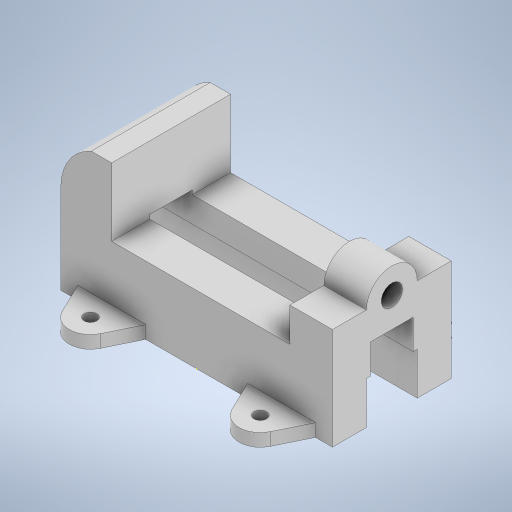
# Autodesk Inventor part: Pieza5-Tarea1
Saved by Autodesk Inventor 2024 (Build 280153000, 153)
## iProperties
Created: 2024-02-16
Part Number: Pieza5-Tarea1
Material: Genérico
Document SubType Name: Modeling
Designer: Diegolap
Density: 1 g/cm^3
Appearance: Valor por defecto
Mass: 816.406 g
Surface Area: 1054.14 cm^2
Volume: 816.406 cm^3
Author: Diegolap
Autodesk Inventor part; units mm, degrees
ref_plane "YZ Plane" through (0, 0, 0) normal (1, 0, 0) x (0, 1, 0)
ref_plane "XZ Plane" through (0, 0, 0) normal (0, 1, 0) x (-1, 0, 0)
ref_plane "XY Plane" through (0, 0, 0) normal (0, 0, 1) x (1, 0, 0)
sketch "Boceto1" plane through (0, 0, 0) normal (0, 1, 0) x (-1, 0, 0)
  line L0 (-101.6, 44.45) -> (101.6, 44.45)
  line L1 (101.6, 44.45) -> (101.6, -44.45)
  line L2 (101.6, -44.45) -> (-101.6, -44.45)
  line L3 (-101.6, -44.45) -> (-101.6, 44.45)
  line L4 (-101.6, 44.45) -> (101.6, -44.45) construction
  line L5 (101.6, 44.45) -> (-101.6, -44.45) construction
  point P0 (0, 0)
  dimension "d0" = 88.9
  dimension "d1" = 203.2
  constraints: 12 end point, 2 midpoint, 2 parallel, 1 horizontal, 1 perpendicular
  measures "d0" distance of L0.end L1.end
  measures "d1" distance of L0.start L0.end
extrude "Extrusión1" add sketch "Boceto1" along normal blind 50.8
sketch "Boceto2" plane through (0, 50.8, 0) normal (0, 1, 0) x (1, 0, 0)
  line L0 (101.6, 44.45) -> (-101.6, 44.45) projected
  line L1 (101.6, 44.45) -> (69.85, 44.45)
  line L2 (69.85, 44.45) -> (69.85, -44.45)
  line L3 (69.85, -44.45) -> (101.6, -44.45)
  line L4 (101.6, -44.45) -> (101.6, 44.45)
  point P0 (0, 0)
  dimension "d4" = 88.9
  dimension "d5" = 31.75
  constraints: 8 end point, 2 parallel, 1 horizontal, 1 perpendicular
  measures "d4" distance of L1.end L2.end
  measures "d5" distance of L2.end L3.end
extrude "Extrusión2" add sketch "Boceto2" along normal blind 25.4
sketch "Boceto3" plane through (101.6, 0, 44.45) normal (1, 0, 0) x (0, 0, -1)
  line L0 (0, 0) -> (0, 76.2) projected
  line L1 (0, 76.2) -> (88.9, 76.2) projected
  line L2 (0, 76.2) -> (88.9, 76.2)
  circle A0 centre (44.45, 76.2) radius 19.05
  circle A1 centre (44.45, 76.2) radius 7.9375
  point P0 (44.45, 0)
  dimension "d8" = 38.1
  dimension "d9" = 15.875
  constraints: 2 centre point, 2 end point, 1 coincident, 1 collinear, 1 midpoint
  measures "d8" diameter of A0
  measures "d9" diameter of A1
extrude "Extrusión3" add sketch "Boceto3" against normal blind 31.75 contours A1 L1 A0 | L1 A0 A1
sketch "Boceto4" plane through (101.6, 0, 44.45) normal (1, 0, 0) x (0, 0, -1)
  line L0 (52.3875, 76.2) -> (36.5125, 76.2) projected
  circle A0 centre (44.45, 76.2) radius 7.9375
  point P0 (44.45, 0)
  dimension "d12" = 15.875
  constraints: 1 centre point, 1 midpoint
  measures "d12" diameter of A0
extrude "Extrusión4" cut sketch "Boceto4" against normal blind 31.75
sketch "Boceto5" plane through (0, 50.8, 0) normal (0, 1, 0) x (1, 0, 0)
  line L0 (-101.6, -44.45) -> (101.6, -44.45) projected
  line L1 (-101.6, -44.45) -> (-63.5, -44.45)
  line L2 (-63.5, -44.45) -> (-63.5, 44.45)
  line L3 (-63.5, 44.45) -> (-101.6, 44.45)
  line L4 (-101.6, 44.45) -> (-101.6, -44.45)
  point P0 (0, 0)
  dimension "d15" = 38.1
  dimension "d16" = 88.9
  constraints: 8 end point, 2 parallel, 1 horizontal, 1 perpendicular
  measures "d15" distance of L2.end L3.end
  measures "d16" distance of L1.end L2.end
extrude "Extrusión5" add sketch "Boceto5" along normal blind 50.8
sketch "Boceto6" plane through (-101.6, 0, 44.45) normal (0, 0, 1) x (1, 0, 0)
  line L0 (0, 0) -> (0, 66.675)
  line L1 (0, 0) -> (0, 101.6) projected
  line L2 (38.1, 50.8) -> (38.1, 101.6) projected
  circle A0 centre (38.1, 66.675) radius 38.1
  line L3 (0, 66.675) -> (0, 101.6)
  line L4 (0, 101.6) -> (22.8732, 101.6)
  line L5 (0, 101.6) -> (38.1, 101.6) projected
  point P0 (101.6, 0)
  dimension "d20" = 76.2
  dimension "d19" = 66.675
  constraints: 6 end point, 3 point on line, 1 collinear, 3 other
  measures "d19" distance of L0.end L0.start
extrude "Extrusión6" cut sketch "Boceto6" against normal blind 101.6 contours L1 L4 A0
sketch "Boceto7" plane through (101.6, 0, 44.45) normal (1, 0, 0) x (0, 0, -1)
  line L0 (25.4, -31.75) -> (63.5, -31.75)
  line L1 (63.5, -31.75) -> (63.5, 31.75)
  line L2 (63.5, 31.75) -> (25.4, 31.75)
  line L3 (25.4, 31.75) -> (25.4, -31.75)
  line L4 (25.4, -31.75) -> (63.5, 31.75) construction
  line L5 (63.5, -31.75) -> (25.4, 31.75) construction
  line L6 (60.325, 53.975) -> (28.575, 53.975)
  line L7 (28.575, 53.975) -> (28.575, 31.75)
  line L8 (60.325, 31.75) -> (60.325, 53.975)
  line L9 (44.45, 31.75) -> (60.325, 53.975) construction
  line L10 (44.45, 31.75) -> (28.575, 53.975) construction
  point P0 (44.45, 0)
  dimension "d23" = 63.5
  dimension "d24" = 38.1
  dimension "d25" = 31.75
  dimension "d26" = 22.225
  dimension "d27" = 22.225
  dimension "d28" = 90
  dimension "d29" = 90
  constraints: 22 end point, 4 midpoint, 3 parallel, 2 point on line, 1 horizontal, 1 perpendicular
  measures "d23" distance of L0.end L1.end
  measures "d24" distance of L1.end L2.end
  measures "d25" distance of L6.start L6.end
  measures "d26" distance of L8.start L6.start
  measures "d27" distance of L6.end L7.end
  measures "d28" angle of L7 L6
  measures "d29" angle of L8 L6
extrude "Extrusión7" cut sketch "Boceto7" against normal blind 254
sketch "Boceto8" plane through (-101.6, 0, 44.45) normal (0, 0, 1) x (1, 0, 0)
  point P0 (101.6, 0)
sketch "Boceto9" plane through (0, 0, 0) normal (0, -1, 0) x (1, 0, 0)
  line L0 (-101.6, 44.45) -> (101.6, 44.45) projected
  line L1 (101.6, 44.45) -> (88.9, 44.45)
  line L2 (88.9, 44.45) -> (38.1, 44.45)
  line L3 (63.5, 44.45) -> (63.5, 60.325)
  circle A0 centre (63.5, 60.325) radius 4.7625
  circle A1 centre (63.5, 60.325) radius 15.875
  line L4 (38.1, 44.45) -> (49.2303, 67.2815)
  line L5 (88.9, 44.45) -> (77.7697, 67.2815)
  point P0 (0, 0)
  dimension "d32" = 12.7
  dimension "d33" = 50.8
  dimension "d34" = 15.875
  dimension "d35" = 9.525
  dimension "d36" = 31.75
  constraints: 10 end point, 2 centre point, 2 coincident, 2 point on circle, 2 point on line, 2 tangent, 1 midpoint, 1 vertical
  measures "d32" distance of L1.end L0.end
  measures "d33" distance of L2.end L1.end
  measures "d34" distance of L3.start L3.end
  measures "d35" diameter of A0
  measures "d36" diameter of A1
extrude "Extrusión8" add sketch "Boceto9" against normal blind 9.525
mirror "Simetría1" about plane through (0, 0, 0) normal (1, 0, 0) of "Extrusión8"
mirror "Simetría2" about plane through (0, 0, 0) normal (0, 0, 1) of "Extrusión8", "Simetría1"
